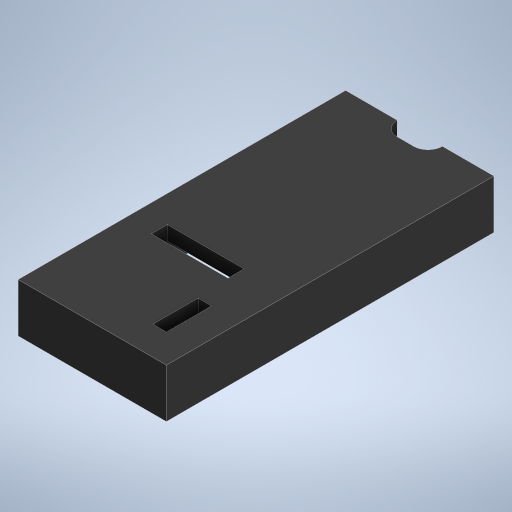
# Autodesk Inventor part: RadioMountCover
Saved by Autodesk Inventor 2024 (Build 280153000, 153)
## iProperties
Created: 2023-08-23
Part Number: RadioMountCover
Material: Rubber, Silicone
Document SubType Name: Modeling
Designer: 18179
Density: 1.25 g/cm^3
Appearance: Rubber - Black
Author: 18179
Autodesk Inventor part; units mm, degrees
ref_plane "YZ Plane" through (0, 0, 0) normal (1, 0, 0) x (0, 1, 0)
ref_plane "XZ Plane" through (0, 0, 0) normal (0, 1, 0) x (-1, 0, 0)
ref_plane "XY Plane" through (0, 0, 0) normal (0, 0, 1) x (1, 0, 0)
sketch "Sketch1" plane through (0, 0, 0) normal (0, 1, 0) x (-1, 0, 0)
  line L0 (0, 0) -> (26.416, 0)
  line L1 (26.416, 0) -> (26.416, -66.04)
  line L2 (26.416, -66.04) -> (0, -66.04)
  line L3 (0, -66.04) -> (0, 0)
  line L4 (29.591, -69.215) -> (29.591, 3.175)
  line L5 (29.591, 3.175) -> (-3.175, 3.175)
  line L6 (-3.175, 3.175) -> (-3.175, -69.215)
  line L7 (-3.175, -69.215) -> (29.591, -69.215)
  line L8 (13.208, -69.215) -> (18.208, -69.215)
  line L9 (18.208, -69.215) -> (18.208, -66.04)
  line L10 (18.208, -66.04) -> (13.208, -66.04)
  line L11 (13.208, -66.04) -> (13.208, -69.215)
  line L12 (13.208, -66.04) -> (8.208, -66.04)
  line L13 (8.208, -66.04) -> (8.208, -69.215)
  line L14 (8.208, -69.215) -> (13.208, -69.215)
  line L15 (13.208, -69.215) -> (13.208, -66.04)
  point P0 (18.208, -69.215)
  point P1 (8.208, -66.04)
  dimension "d0" = 26.416
  dimension "d1" = 66.04
  dimension "d2" = 3.175
  dimension "d3" = 5
  dimension "d4" = 5
  constraints: 32 end point, 8 parallel, 4 perpendicular, 3 horizontal, 2 point on line, 1 midpoint, 3 other
  measures "d0" distance of L1.end L2.end
  measures "d1" distance of L0.end L1.end
  measures "d2" distance between parallel lines of L1 L4
  measures "d3" distance of L10.end L9.end
  measures "d4" distance of L14.end L13.end
extrude "Extrusion1" add sketch "Sketch1" along normal blind 7.62 contours L3 L2 L13 L7 L6 L5 L4 L9 L1 L0
sketch "Sketch2" plane through (0, 7.62, 0) normal (0, 1, 0) x (1, 0, 0)
  line L0 (-26.416, 0) -> (-26.416, 66.04) projected
  line L1 (-26.416, 0) -> (0, 0)
  line L2 (0, 0) -> (0, 66.04)
  line L3 (0, 66.04) -> (-26.416, 66.04)
  line L4 (-26.416, 66.04) -> (-26.416, 0)
  line L5 (-3.175, 3.175) -> (-23.241, 3.175)
  line L6 (-23.241, 3.175) -> (-23.241, 62.865)
  line L7 (-23.241, 62.865) -> (-3.175, 62.865)
  line L8 (-3.175, 62.865) -> (-3.175, 3.175)
  line L9 (-3.175, 3.175) -> (-6.175, 3.175)
  line L10 (-6.175, 3.175) -> (-6.175, 13.175)
  line L11 (-6.175, 13.175) -> (-3.175, 13.175)
  line L12 (-3.175, 13.175) -> (-3.175, 3.175)
  line L13 (-26.416, 66.04) -> (-18.208, 66.04) projected
  line L14 (0, 66.04) -> (0, 0) projected
  line L15 (-6.175, 13.175) -> (-6.675, 13.175)
  line L16 (-6.675, 13.175) -> (-6.675, 20.287)
  line L17 (-6.675, 20.287) -> (-6.175, 20.287)
  line L18 (-6.175, 20.287) -> (-6.175, 13.175)
  line L19 (-6.675, 20.287) -> (-23.6463, 20.287)
  line L20 (-23.6463, 20.287) -> (-23.6463, 23.8513)
  line L21 (-23.6463, 23.8513) -> (-6.675, 23.8513)
  line L22 (-6.675, 23.8513) -> (-6.675, 20.287)
  point P0 (-26.416, 66.04)
  dimension "d8" = 3.175
  dimension "d9" = 3
  dimension "d10" = 10
  dimension "d11" = 0.5
  dimension "d12" = 7.112
  constraints: 40 end point, 10 parallel, 5 perpendicular, 4 horizontal, 2 collinear, 3 other
  measures "d8" distance between parallel lines of L1 L5
  measures "d9" distance of L10.end L11.end
  measures "d10" distance of L9.end L10.end
  measures "d11" distance of L16.end L17.end
  measures "d12" distance of L15.end L16.end
extrude "Extrusion2" add sketch "Sketch2" along normal blind 3.175 contours L0 L3 L2 L1 | L5 L6 L19 L16 L15 L10 | L11 L18 L17 L22 L21 L6 L7 L8 | L15 L16 L17 L18
sketch "Sketch3" plane through (0, 7.62, 0) normal (0, 1, 0) x (1, 0, 0)
  line L0 (-26.416, 66.04) -> (-18.208, 66.04) projected
  line L1 (-18.208, 66.04) -> (-18.208, 69.215) projected
  line L2 (-18.208, 69.215) -> (-29.591, 69.215) projected
  line L3 (-29.591, 69.215) -> (-29.591, -3.175) projected
  line L4 (-29.591, -3.175) -> (3.175, -3.175) projected
  line L5 (3.175, -3.175) -> (3.175, 69.215) projected
  line L6 (3.175, 69.215) -> (-8.208, 69.215) projected
  line L7 (-8.208, 69.215) -> (-8.208, 66.04) projected
  line L8 (-8.208, 66.04) -> (0, 66.04) projected
  line L9 (0, 66.04) -> (0, 0) projected
  line L10 (0, 0) -> (-26.416, 0) projected
  line L11 (-26.416, 0) -> (-26.416, 66.04) projected
extrude "Extrusion3" add sketch "Sketch3" along normal blind 3.175
fillet "Fillet1" radius 3.175 2 edges at (-18.208, 9.2075, -66.04) (-8.208, 9.2075, -66.04)
sketch "Sketch4" plane through (0, 0, 0) normal (0, -1, 0) x (1, 0, 0)
  line L0 (0, 0) -> (-26.416, 0) projected
  line L1 (-26.416, -66.04) -> (-18.208, -66.04) projected
  line L2 (0, 0) -> (-26.416, 0)
  line L3 (-26.416, 0) -> (-26.416, -66.04)
  line L4 (-26.416, -66.04) -> (0, -66.04)
  line L5 (0, -66.04) -> (0, 0)
  line L6 (0.254, 0.254) -> (-26.67, 0.254)
  line L7 (-26.67, 0.254) -> (-26.67, -66.294)
  line L8 (-26.67, -66.294) -> (0.254, -66.294)
  line L9 (0.254, -66.294) -> (0.254, 0.254)
  dimension "d18" = 0.254
  constraints: 16 end point, 4 parallel, 2 perpendicular, 1 horizontal, 3 other
  measures "d18" distance between parallel lines of L5 L9
extrude "Extrusion4" cut sketch "Sketch4" against normal up to surface (7.62 mm away) contours L5 L4 L1 L3 L0 | L9 L8 L7 L6
body "Solid1"
